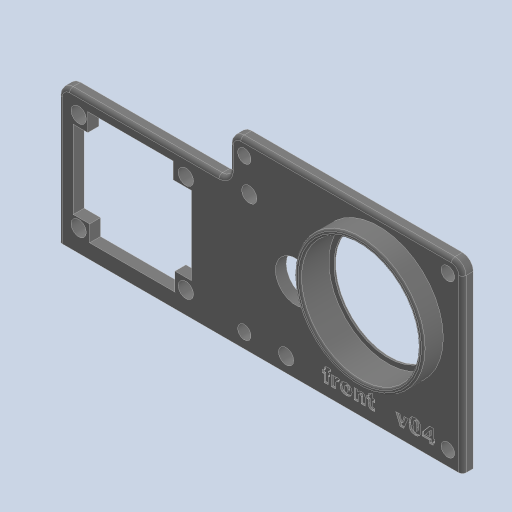
# Autodesk Inventor part: door_front_04
Saved by Autodesk Inventor 2024.4 (Build 284460030, 460C)
## iProperties
Created: 2026-07-13
Part Number: door_front_04
Material: Generic
Document SubType Name: Modeling
Designer: tooles01
Density: 1 g/cm^3
Appearance: Gray
d0: 3.000 mm
d3: 32.500 mm
d4: 35.500 mm
d11: 29.750 mm
d14: 3.700 mm
d0_1: 36.000 mm
d3_1: 4.900 mm
d4_1: 3.000 mm
d5_1: 10.000 mm
d6_1: 2.000 mm
d7: 2.000 mm
d21: 30.000 mm
d22: 64.000 mm
d23: 4.000 mm
d24: 4.000 mm
d25: 4.000 mm
d26: 4.200 mm
d27: 35.000 mm
d28: 3.000 mm
d29: 4.900 mm
d32: 6.500 mm
d33: 2.000 mm
d34: 2.000 mm
d35: 10.000 mm
d37: 36.000 mm
d38: 2.000 mm
d39: 4.900 mm
d41: 4.200 mm
d68: 20.000 mm
d72: 40.000 mm
d73: 0.500 mm
d75: 5.000 mm
door_diameter: 36.000 mm
axle_width: 4.900 mm
axle_height: 3.100 mm
handle_height: 10.000 mm
spacing_height: 2.000 mm
spacing_width: 2.000 mm
door_diameter_1: 36.000 mm
handle_height_1: 10.000 mm
spacing_width_1: 2.000 mm
door_spacing_width_1: 2.000 mm
door_handle_height_1: 10.000 mm
door_door_diameter_1: 36.000 mm
door_axle_width_1: 4.900 mm
door_spacing_height_1: 2.000 mm
door_axle_width_2: 4.900 mm
door_axle_height_1: 3.100 mm
door_spacing_height_2: 2.000 mm
d76: 4.000 mm
d77: 9.200 mm
d78: 1.000 mm
M3_heatset: 4.200 mm
tube_cover_length: 8.500 mm
tube_stopper_thickness: 0.500 mm
x_e1: 0.00 deg
x_e2: 0.00 deg
x_e3: 0.00 deg
x_e4: 0.00 deg
x_f2: 1.000 mm
x_f3: 0.500 mm
x_0: 1.000 ul
x_f1: 3.000 mm
length_of_tube_pressfit: 8.000 mm
M3_through_hole: 3.700 mm
motor_diameter: 28.000 mm
d137: 90.00 deg
d139: 3.500 mm
d169: 3.000 mm
d170: 0.00 deg
d171: 32.000 mm
d172: 27.000 mm
d173: 2.000 mm
d174: 3.000 mm
d175: 2.500 mm
d176: 34.500 mm
d177: 29.500 mm
d178: 4.200 mm
d185: 3.000 mm
d186: 2.500 mm
d187: 1.000 mm
d188: 3.500 mm
d189: 3.000 mm
d190: 2.500 mm
d191: 1.000 mm
d192: 1.000 mm
d193: 2.500 mm
d194: 2.000 mm
d195: 0.500 mm
d196: 50.000 mm
d198: 41.000 mm
d199: 4.000 mm
d200: 23.000 mm
d201: 6.000 mm
d202: 3.000 mm
d203: 3.000 mm
d204: 3.000 mm
d205: 3.000 mm
d206: 3.000 mm
Author: tooles01
Autodesk Inventor part; units mm, degrees
ref_plane "YZ Plane" through (0, 0, 0) normal (1, 0, 0) x (0, 1, 0)
ref_plane "XZ Plane" through (0, 0, 0) normal (0, 1, 0) x (-1, 0, 0)
ref_plane "XY Plane" through (0, 0, 0) normal (0, 0, 1) x (1, 0, 0)
derived "door_03.ipt"
sketch "Sketch1: base" plane through (0, 0, 0) normal (0, 0, 1) x (1, 0, 0)
  line L0 (-41, 50) -> (23, 50)
  line L1 (23, 50) -> (23, 0)
  line L2 (23, 0) -> (-41, 0)
  line L3 (-41, 0) -> (-41, 50)
  circle A0 centre (0, 30) radius 16.25
  line L4 (-37, 46) -> (19, 46) construction
  line L5 (19, 46) -> (19, 4) construction
  line L6 (19, 4) -> (-37, 4) construction
  line L7 (-37, 4) -> (-37, 46) construction
  point P0 (0, 0)
  dimension "d3" = 32.5
  dimension "d21" = 30
  dimension "d22" = 64
  dimension "d23" = 4
  dimension "d24" = 4
  dimension "d25" = 4
  dimension "d68" = 20
  dimension "d196" = 50
  dimension "d198" = 41
  dimension "d199" = 4
  dimension "d200" = 23
  constraints: 16 end point, 6 perpendicular, 4 coincident, 2 horizontal, 1 centre point, 1 point on line, 1 vertical alignment
  measures "d3" diameter of A0
  measures "d21" distance from line of L2 A0.centre
  measures "d22" distance of L1.end L2.end
  measures "d23" distance between parallel lines of L2 L6
  measures "d24" distance between parallel lines of L3 L7
  measures "d25" distance between parallel lines of L0 L4
  measures "d68" distance from line of L0 A0.centre
  measures "d196" distance between parallel lines of L0 L2
  measures "d198" distance from line of L3 A0.centre
  measures "d199" distance between parallel lines of L1 L5
  measures "d200" distance from line of L1 A0.centre
sketch "Sketch2: tube cover/stopper" plane through (0, 0, 0) normal (0, 0, 1) x (1, 0, 0)
  circle A0 centre (0, 30) radius 17.75
  circle A1 centre (0, 30) radius 14.875
  circle A2 centre (0, 30) radius 16.25 projected
  point P0 (0, 0)
  dimension "d4" = 35.5
  dimension "d11" = 29.75
  constraints: 3 coincident, 2 centre point
  measures "d4" diameter of A0
  measures "d11" diameter of A1
sketch "Sketch3: motor & door footprint" plane through (0, 0, 0) normal (0, 0, 1) x (1, 0, 0)
  circle A0 centre (-35.6404, 37.5002) radius 2.1 construction
  circle A1 centre (-25.5048, 4) radius 2.1 construction
  line L0 (-35.6404, 37.5002) -> (-25.5048, 4) construction
  line L1 (-22.0934, 25.8752) -> (-20.6745, 21.1852)
  line L2 (-20.6745, 21.1852) -> (-23.6416, 20.2874)
  line L3 (-23.6416, 20.2874) -> (-25.0606, 24.9775)
  line L4 (-25.0606, 24.9775) -> (-22.0934, 25.8752)
  line L5 (-24.3511, 22.6325) -> (-30.5726, 20.7501) construction
  line L6 (-27.5541, 26.3126) -> (-24.9767, 17.7939)
  line L7 (-24.9767, 17.7939) -> (-15.4052, 20.6899)
  line L8 (-17.9826, 29.2085) -> (-27.5541, 26.3126)
  circle A2 centre (0, 30) radius 18
  line L9 (0, 30) -> (-26.2654, 22.0533) construction
  circle A3 centre (0, 30) radius 16.25 construction
  circle A4 centre (-29.7862, 45.9488) radius 18 construction
  line L10 (-28.9947, 27.9663) -> (-26.0988, 18.3948) construction
  line L11 (-26.0988, 18.3948) -> (-17.5802, 20.9721) construction
  line L12 (-17.5802, 20.9721) -> (-20.4761, 30.5436) construction
  line L13 (-20.9714, 25.2744) -> (-25.6614, 23.8554) construction
  line L14 (-25.6614, 23.8554) -> (-24.7637, 20.8882) construction
  line L15 (-24.7637, 20.8882) -> (-20.0736, 22.3072) construction
  line L16 (-20.0736, 22.3072) -> (-20.9714, 25.2744) construction
  line L17 (-29.7862, 45.9488) -> (-21.8395, 19.6834) construction
  circle A5 centre (-22.8675, 23.0813) radius 2.45 construction
  circle A6 centre (-30.5726, 20.7501) radius 14 construction
  arc A7 (-28.8548, 2.9864) -> (-22.1547, 5.0136) centre (-25.5048, 4) ccw construction
  line L18 (-29.9971, 6.7619) -> (-28.8548, 2.9864) construction
  line L19 (-23.297, 8.7891) -> (-22.1547, 5.0136) construction
  line L20 (-29.9971, 0.5) -> (-23.297, 0.5) construction
  arc A8 (-32.2904, 38.5138) -> (-38.9905, 36.4867) centre (-35.6404, 37.5002) ccw construction
  line L21 (-38.9905, 36.4867) -> (-37.8482, 32.7111) construction
  line L22 (-32.2904, 38.5138) -> (-31.1481, 34.7383) construction
  line L23 (-36.2123, 41.0002) -> (-30.5422, 41.0002) construction
  point P0 (0, 0)
  point P1 (-21.3839, 23.5302)
  point P2 (-22.4187, 21.5977)
  point P3 (-22.158, 20.7363)
  point P4 (-20.5225, 23.7908)
  dimension "d26" = 4.2
  dimension "d27" = 34.9999
  dimension "door_axle_height_1" = 3.1
  dimension "door_axle_width_1" = 4.9
  dimension "d32" = 6.5
  dimension "door_spacing_height_1" = 2
  dimension "door_spacing_width_1" = 2
  dimension "door_handle_height_1" = 10
  dimension "door_door_diameter_1" = 36
  dimension "door_spacing_height_2" = 2
  dimension "door_axle_width_2" = 4.9
  dimension "motor_diameter" = 28
  dimension "d137" = 90
  dimension "d139" = 3.5
  dimension "d195" = 0.5
  constraints: 48 end point, 14 point on circle, 9 parallel, 8 centre point, 8 coincident, 8 midpoint, 8 perpendicular, 6 equal length, 6 tangent, 4 point on line, 3 equal radius, 2 horizontal, 2 vertical alignment, 1 collinear
  measures "d26" diameter of A0
  measures "d27" distance of L0.start L0.end
  measures "door_axle_height_1" distance of L3.end L1.start
  measures "door_axle_width_1" distance of L1.start L1.end
  measures "d32" distance from line of A0.centre L3
  measures "door_spacing_height_1" distance between parallel lines of L6 L3
  measures "door_spacing_width_1" distance between parallel lines of L8 L4
  measures "door_handle_height_1" distance of L8.start L6.start
  measures "door_door_diameter_1" diameter of A2
  measures "door_spacing_height_2" distance between parallel lines of L11 L15
  measures "door_axle_width_2" diameter of A5
  measures "motor_diameter" diameter of A6
  measures "d137" angle of L9 L17
  measures "d139" radius of A7
  measures "d195" distance from line of point (0, 0) L20
sketch "Sketch4: holes for motor mount" plane through (0, 0, 0) normal (0, 0, 1) x (1, 0, 0)
  circle A0 centre (-22.8675, 23.0813) radius 2.45 construction
  circle A1 centre (-22.8675, 23.0813) radius 5.6
  circle A2 centre (-22.8675, 23.0813) radius 4.6 construction
  point P0 (0, 0)
  point P1 (-35.6404, 37.5002)
  point P2 (-25.5048, 4)
  dimension "d77" = 9.2
  dimension "d78" = 1
  constraints: 2 centre point, 2 coincident
  measures "d77" diameter of A2
  measures "d78" radial gap between concentric circles of A1 A2
sketch "Sketch: space for PCB footprint" plane through (0, 0, 0) normal (0, 0, 1) x (1, 0, 0)
  line L0 (-56.0726, 4) -> (-79.5726, 4)
  line L1 (-80.0726, 35) -> (-56.5726, 35)
  line L2 (-56.5726, 30.5) -> (-51.5726, 30.5)
  line L3 (-51.5726, 30.5) -> (-51.5726, 9)
  line L4 (-51.5726, 9) -> (-56.0726, 9)
  line L5 (-80.0726, 30) -> (-84.0726, 30)
  line L6 (-84.0726, 30) -> (-84.0726, 8.5)
  line L7 (-84.0726, 8.5) -> (-79.5726, 8.5)
  line L8 (-56.0726, 9) -> (-56.0726, 4)
  line L9 (-79.5726, 8.5) -> (-79.5726, 4)
  line L10 (-88.0726, 38) -> (-41, 38)
  line L11 (-41, 0) -> (-88.0726, 0)
  line L12 (-88.0726, 0) -> (-88.0726, 38)
  line L13 (-41, 0) -> (-41, 50) projected
  line L14 (23, 0) -> (-41, 0) projected
  line L15 (-23.297, 8.7891) -> (-22.1547, 5.0136) construction
  arc A0 (-28.8548, 2.9864) -> (-22.1547, 5.0136) centre (-25.5048, 4) ccw construction
  line L16 (-29.9971, 6.7619) -> (-28.8548, 2.9864) construction
  circle A1 centre (-30.5726, 20.7501) radius 14 construction
  line L17 (-80.0726, 35) -> (-80.0726, 30)
  line L18 (-56.5726, 35) -> (-56.5726, 30.5)
  line L19 (-85.0726, 35) -> (-50.5726, 35) construction
  line L20 (-50.5726, 35) -> (-50.5726, 3) construction
  line L21 (-50.5726, 3) -> (-85.0726, 3) construction
  line L22 (-85.0726, 3) -> (-85.0726, 35) construction
  circle A2 centre (-82.5726, 33) radius 1.5 construction
  circle A3 centre (-53.0726, 33) radius 1.5 construction
  circle A4 centre (-82.5726, 6) radius 1.5 construction
  circle A5 centre (-53.0726, 6) radius 1.5 construction
  line L23 (-82.5726, 33) -> (-53.0726, 33) construction
  line L24 (-53.0726, 33) -> (-53.0726, 6) construction
  line L25 (-44.5726, 38) -> (-44.5726, 0) construction
  point P0 (0, 0)
  point P1 (-61.5, 13)
  dimension "d171" = 32
  dimension "d172" = 27
  dimension "d173" = 2
  dimension "d174" = 3
  dimension "d175" = 2.5
  dimension "d176" = 34.5
  dimension "d177" = 29.5
  dimension "d185" = 3
  dimension "d186" = 2.5
  dimension "d187" = 1
  dimension "d188" = 3.5
  dimension "d189" = 3
  dimension "d190" = 2.5
  dimension "d191" = 1
  dimension "d192" = 1
  dimension "d193" = 2.5
  dimension "d194" = 2
  dimension "d201" = 6
  dimension "d202" = 3
  dimension "d203" = 3
  dimension "d204" = 3
  dimension "d205" = 3
  dimension "d206" = 3
  constraints: 44 end point, 16 perpendicular, 4 centre point, 3 coincident, 3 equal radius, 3 horizontal, 3 point on line, 1 collinear, 1 horizontal alignment, 1 tangent, 1 vertical, 1 vertical alignment
  measures "d171" distance of L21.end L19.start
  measures "d172" distance of A4.centre A2.centre
  measures "d173" distance between parallel lines of L19 L23
  measures "d174" diameter of A2
  measures "d175" distance from line of L22 A2.centre
  measures "d176" distance of L19.start L19.end
  measures "d177" distance of L23.start L23.end
  measures "d185" distance from line of A4.centre L9
  measures "d186" distance from line of A4.centre L7
  measures "d187" distance between parallel lines of L21 L0
  measures "d188" distance from line of L18 A3.centre
  measures "d189" distance from line of L5 A2.centre
  measures "d190" distance from line of L17 A2.centre
  measures "d191" distance between parallel lines of L20 L3
  measures "d192" distance between parallel lines of L22 L6
  measures "d193" distance from line of A3.centre L2
  measures "d194" distance from line of L1 A3.centre
  measures "d201" distance between parallel lines of L25 L20
  measures "d202" distance between parallel lines of L12 L22
  measures "d203" distance between parallel lines of L11 L21
  measures "d204" distance between parallel lines of L10 L19
  measures "d205" distance from line of L8 A5.centre
  measures "d206" distance from line of L4 A5.centre
sketch "Sketch6: text" plane through (0, 0, 0) normal (0, 0, 1) x (1, 0, 0)
  line L0 (-20, 7) -> (20, 7) construction
  line L1 (20, 7) -> (20, 3) construction
  line L2 (20, 3) -> (-20, 3) construction
  line L3 (-20, 3) -> (-20, 7) construction
  line L4 (-13.9634, 5.8989) -> (-13.4321, 5.8989)
  line L5 (-13.4321, 5.8989) -> (-13.4321, 5.0866)
  line L6 (-13.4321, 5.0866) -> (-13.9634, 5.0866)
  line L7 (-13.9634, 5.0866) -> (-13.9634, 3)
  line L8 (-13.9634, 3) -> (-15.076, 3)
  line L9 (-15.076, 3) -> (-15.076, 5.0866)
  line L10 (-15.076, 5.0866) -> (-15.4918, 5.0866)
  line L11 (-15.4918, 5.0866) -> (-15.4918, 5.8989)
  line L12 (-15.4918, 5.8989) -> (-15.076, 5.8989)
  line L13 (-15.076, 5.8989) -> (-15.076, 6.0298)
  spline S0 degree 2 poles (-15.076, 6.0298) (-15.076, 6.2069) (-14.999, 6.6343) (-14.7911, 6.9038) (-14.41, 7.0693) (-14.0443, 7.0693) knots 0 0 0 1 2 3 4 4 4
  spline S1 degree 2 poles (-14.0443, 7.0693) (-13.7517, 7.0693) (-13.1973, 7) knots 0 0 0 1 1 1
  line L14 (-13.1973, 7) -> (-13.3205, 6.3301)
  spline S2 degree 2 poles (-13.3205, 6.3301) (-13.5168, 6.3609) (-13.64, 6.3609) knots 0 0 0 1 1 1
  spline S3 degree 2 poles (-13.64, 6.3609) (-13.7902, 6.3609) (-13.9211, 6.2608) (-13.948, 6.153) knots 0 0 0 1 2 2 2
  spline S4 degree 2 poles (-13.948, 6.153) (-13.9634, 6.0914) (-13.9634, 5.8989) knots 0 0 0 1 1 1
  line L15 (-13.0125, 5.8989) -> (-11.9731, 5.8989)
  line L16 (-11.9731, 5.8989) -> (-11.9731, 5.4254)
  spline S5 degree 2 poles (-11.9731, 5.4254) (-11.8229, 5.7334) (-11.5034, 5.9644) (-11.2685, 5.9644) knots 0 0 0 1 2 2 2
  spline S6 degree 2 poles (-11.2685, 5.9644) (-11.0221, 5.9644) (-10.7295, 5.8104) knots 0 0 0 1 1 1
  line L17 (-10.7295, 5.8104) -> (-11.0722, 5.0212)
  spline S7 degree 2 poles (-11.0722, 5.0212) (-11.2685, 5.102) (-11.384, 5.102) knots 0 0 0 1 1 1
  spline S8 degree 2 poles (-11.384, 5.102) (-11.6035, 5.102) (-11.7228, 4.9211) knots 0 0 0 1 1 1
  spline S9 degree 2 poles (-11.7228, 4.9211) (-11.8961, 4.667) (-11.8961, 3.9702) knots 0 0 0 1 1 1
  line L18 (-11.8961, 3.9702) -> (-11.8961, 3)
  line L19 (-11.8961, 3) -> (-13.0125, 3)
  line L20 (-13.0125, 3) -> (-13.0125, 5.8989)
  spline S10 degree 2 poles (-10.6756, 4.4398) (-10.6756, 5.1059) (-9.7825, 5.9644) (-9.0202, 5.9644) knots 0 0 0 1 2 2 2
  spline S11 degree 2 poles (-9.0202, 5.9644) (-8.1501, 5.9644) (-7.7074, 5.4601) knots 0 0 0 1 1 1
  spline S12 degree 2 poles (-7.7074, 5.4601) (-7.3494, 5.052) (-7.3494, 4.4591) knots 0 0 0 1 1 1
  spline S13 degree 2 poles (-7.3494, 4.4591) (-7.3494, 3.7892) (-8.2348, 2.9346) (-9.0164, 2.9346) knots 0 0 0 1 2 2 2
  spline S14 degree 2 poles (-9.0164, 2.9346) (-9.717, 2.9346) (-10.1482, 3.2887) knots 0 0 0 1 1 1
  spline S15 degree 2 poles (-10.1482, 3.2887) (-10.6756, 3.7276) (-10.6756, 4.4398) knots 0 0 0 1 1 1
  spline S16 degree 2 poles (-9.563, 4.4437) (-9.563, 4.0549) (-9.2512, 3.6853) (-9.0125, 3.6853) knots 0 0 0 1 2 2 2
  spline S17 degree 2 poles (-9.0125, 3.6853) (-8.7738, 3.6853) (-8.4658, 4.051) (-8.4658, 4.4552) knots 0 0 0 1 2 2 2
  spline S18 degree 2 poles (-8.4658, 4.4552) (-8.4658, 4.8287) (-8.7777, 5.1983) (-9.0048, 5.1983) knots 0 0 0 1 2 2 2
  spline S19 degree 2 poles (-9.0048, 5.1983) (-9.2474, 5.1983) (-9.563, 4.8248) (-9.563, 4.4437) knots 0 0 0 1 2 2 2
  line L21 (-6.8104, 5.8989) -> (-5.7748, 5.8989)
  line L22 (-5.7748, 5.8989) -> (-5.7748, 5.4254)
  spline S20 degree 2 poles (-5.7748, 5.4254) (-5.5438, 5.718) (-5.0664, 5.9644) (-4.7276, 5.9644) knots 0 0 0 1 2 2 2
  spline S21 degree 2 poles (-4.7276, 5.9644) (-4.2656, 5.9644) (-3.7459, 5.4139) (-3.7459, 4.8441) knots 0 0 0 1 2 2 2
  line L23 (-3.7459, 4.8441) -> (-3.7459, 3)
  line L24 (-3.7459, 3) -> (-4.8624, 3)
  line L25 (-4.8624, 3) -> (-4.8624, 4.5938)
  spline S22 degree 2 poles (-4.8624, 4.5938) (-4.8624, 4.8672) (-5.0626, 5.0943) (-5.2474, 5.0943) knots 0 0 0 1 2 2 2
  spline S23 degree 2 poles (-5.2474, 5.0943) (-5.4475, 5.0943) (-5.6978, 4.7902) (-5.6978, 4.3936) knots 0 0 0 1 2 2 2
  line L26 (-5.6978, 4.3936) -> (-5.6978, 3)
  line L27 (-5.6978, 3) -> (-6.8104, 3)
  line L28 (-6.8104, 3) -> (-6.8104, 5.8989)
  line L29 (-1.7401, 7) -> (-1.7401, 5.8989)
  line L30 (-1.7401, 5.8989) -> (-1.128, 5.8989)
  line L31 (-1.128, 5.8989) -> (-1.128, 5.0866)
  line L32 (-1.128, 5.0866) -> (-1.7401, 5.0866)
  line L33 (-1.7401, 5.0866) -> (-1.7401, 4.0587)
  spline S24 degree 2 poles (-1.7401, 4.0587) (-1.7401, 3.8739) (-1.7055, 3.8123) knots 0 0 0 1 1 1
  spline S25 degree 2 poles (-1.7055, 3.8123) (-1.6516, 3.7199) (-1.513, 3.7199) knots 0 0 0 1 1 1
  spline S26 degree 2 poles (-1.513, 3.7199) (-1.3898, 3.7199) (-1.1704, 3.7892) knots 0 0 0 1 1 1
  line L34 (-1.1704, 3.7892) -> (-1.0895, 3.0231)
  spline S27 degree 2 poles (-1.0895, 3.0231) (-1.5014, 2.9346) (-1.8595, 2.9346) knots 0 0 0 1 1 1
  spline S28 degree 2 poles (-1.8595, 2.9346) (-2.2714, 2.9346) (-2.6641, 3.1463) (-2.8527, 3.5813) (-2.8527, 4.0664) knots 0 0 0 1 2 3 3 3
  line L35 (-2.8527, 4.0664) -> (-2.8527, 5.0866)
  line L36 (-2.8527, 5.0866) -> (-3.2608, 5.0866)
  line L37 (-3.2608, 5.0866) -> (-3.2608, 5.8989)
  line L38 (-3.2608, 5.8989) -> (-2.8527, 5.8989)
  line L39 (-2.8527, 5.8989) -> (-2.8527, 6.4302)
  line L40 (-2.8527, 6.4302) -> (-1.7401, 7)
  line L41 (4.666, 5.8989) -> (5.821, 5.8989)
  line L42 (5.821, 5.8989) -> (6.3869, 4.0626)
  line L43 (6.3869, 4.0626) -> (6.9682, 5.8989)
  line L44 (6.9682, 5.8989) -> (8.0885, 5.8989)
  line L45 (8.0885, 5.8989) -> (6.8566, 3)
  line L46 (6.8566, 3) -> (5.871, 3)
  line L47 (5.871, 3) -> (4.666, 5.8989)
  spline S29 degree 2 poles (8.3041, 5.0173) (8.3041, 6.1569) (9.1242, 7.0693) (9.9634, 7.0693) knots 0 0 0 1 2 2 2
  spline S30 degree 2 poles (9.9634, 7.0693) (10.3677, 7.0693) (10.8835, 6.8691) (11.2108, 6.5496) (11.3994, 6.1992) (11.4572, 5.9644) knots 0 0 0 1 2 3 4 4 4
  spline S31 degree 2 poles (11.4572, 5.9644) (11.5688, 5.5178) (11.5688, 5.0289) knots 0 0 0 1 1 1
  spline S32 degree 2 poles (11.5688, 5.0289) (11.5688, 3.9394) (10.8335, 2.9307) (9.9326, 2.9307) knots 0 0 0 1 2 2 2
  spline S33 degree 2 poles (9.9326, 2.9307) (9.4283, 2.9307) (8.8085, 3.2541) (8.6083, 3.5659) knots 0 0 0 1 2 2 2
  spline S34 degree 2 poles (8.6083, 3.5659) (8.4658, 3.7854) (8.3041, 4.5515) (8.3041, 5.0173) knots 0 0 0 1 2 2 2
  spline S35 degree 2 poles (9.4052, 5.0135) (9.4052, 4.2474) (9.6747, 3.6891) (9.9288, 3.6891) knots 0 0 0 1 2 2 2
  spline S36 degree 2 poles (9.9288, 3.6891) (10.0982, 3.6891) (10.3484, 3.9278) (10.4639, 4.4398) (10.4639, 4.9827) knots 0 0 0 1 2 3 3 3
  spline S37 degree 2 poles (10.4639, 4.9827) (10.4639, 5.7796) (10.1944, 6.3301) (9.9249, 6.3301) knots 0 0 0 1 2 2 2
  spline S38 degree 2 poles (9.9249, 6.3301) (9.6516, 6.3301) (9.4052, 5.7719) (9.4052, 5.0135) knots 0 0 0 1 2 2 2
  line L48 (13.9442, 3.7469) -> (11.9192, 3.7469)
  line L49 (11.9192, 3.7469) -> (11.9192, 4.6631)
  line L50 (11.9192, 4.6631) -> (13.9442, 7.0693)
  line L51 (13.9442, 7.0693) -> (14.9143, 7.0693)
  line L52 (14.9143, 7.0693) -> (14.9143, 4.6092)
  line L53 (14.9143, 4.6092) -> (15.4148, 4.6092)
  line L54 (15.4148, 4.6092) -> (15.4148, 3.7469)
  line L55 (15.4148, 3.7469) -> (14.9143, 3.7469)
  line L56 (14.9143, 3.7469) -> (14.9143, 3)
  line L57 (14.9143, 3) -> (13.9442, 3)
  line L58 (13.9442, 3) -> (13.9442, 3.7469)
  line L59 (13.9442, 4.6092) -> (13.9442, 5.872)
  line L60 (13.9442, 5.872) -> (12.8739, 4.6092)
  line L61 (12.8739, 4.6092) -> (13.9442, 4.6092)
  point P0 (0, 0)
  point P1 (0, 3)
  point P2 (-20, 5)
  dimension "d72" = 40
  dimension "d75" = 5
  dimension "d76" = 4
  constraints: 2 midpoint, 1 horizontal, 1 vertical alignment, 2 other
  measures "d72" distance of L0.start L0.end
  measures "d75" vertical distance of point (0, 0) point (-20, 5)
  measures "d76" distance of L2.end L0.start
extrude "Ex1: base" add sketch "Sketch1: base" along normal blind 3
extrude "Ex2: tube cover" add sketch "Sketch2: tube cover/stopper" along normal blind 8.5 contours A0
extrude "Ex3: tube stopper" add sketch "Sketch2: tube cover/stopper" along normal blind 0.5 contours A2
hole "Hole1: mounting (M3 thru holes)" at (-37, 46, 0) at (19, 46, 0) at (-37, 4, 0) at (19, 4, 0) direction (0, 0, 1) diameter 3.7 end through all
hole "Hole2: motor mount (M3 heat-set)" at (-35.6404, 37.5002, 0) at (-25.5048, 4, 0) direction (0, 0, 1) diameter 4.2 end through all
extrude "Ex4: hole for motor" cut sketch "Sketch4: holes for motor mount" along normal through all both and the other way through all
extrude "Ex: PCB cutout" add sketch "Sketch: space for PCB footprint" along normal blind 3
hole "Hole3: PCB holes (M3 heat-set)" at (-53.0726, 33, 0) at (-82.5726, 33, 0) at (-82.5726, 6, 0) at (-53.0726, 6, 0) direction (0, 0, 1) diameter 4.2 end through all
extrude "Ex5: text" cut sketch "Sketch6: text" against normal blind 0.5 from surface at 3
fillet "Fillet1" radius 3 4 edges at (23, 50, 1.5) (-41, 50, 1.5) (-88.0726, 38, 1.5) (-41, 38, 1.5)
fillet "Fillet2" radius 1 9 edges at (-87.1939, 37.1213, 3) (-88.0726, 17.5, 3) (-41.8787, 38.8787, 3) (-41, 44, 3) (-40.1213, 49.1213, 3) (-9, 50, 3) (22.1213, 49.1213, 3) (23, 23.5, 3) (-64.5363, 38, 3)
fillet "Fillet3" radius 0.5 2 edges at (-16.25, 30, 8.5) (-17.75, 30, 8.5)
equation "\"d24\" = d23"
equation "\"d25\" = d23"
equation "\"M3_heatset\" = 4.2"
equation "\"length_of_tube_pressfit\" = 8"
equation "\"M3_through_hole\" = 3.7"
body "Solid1"
